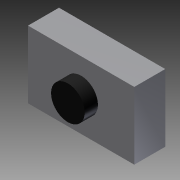
# Autodesk Inventor part: KSR MicroSwitch
Saved by Autodesk Inventor 2012 SP1 (Build 160190100, 190)
## iProperties
Created: 2012-06-05
Part Number: KSR MicroSwitch
Material: Default
Document SubType Name: Modeling
Designer: ding42
Density: 1 g/cm^3
Description: Surface Mount Vertical Tactile Switches
Stock Number: Digi Key Number: 401-1703-1-ND, Manufacturers Number: KSR221GLFS
Catalog Web Link: http://www.digikey.com/catalog/en/partgroup/ksr-series/12817
Author: ding42
Autodesk Inventor part; units mm, degrees
ref_plane "YZ Plane" through (0, 0, 0) normal (1, 0, 0) x (0, 1, 0)
ref_plane "XZ Plane" through (0, 0, 0) normal (0, 1, 0) x (-1, 0, 0)
ref_plane "XY Plane" through (0, 0, 0) normal (0, 0, 1) x (1, 0, 0)
sketch "Sketch1" plane through (0, 0, 0) normal (0, 0, 1) x (1, 0, 0)
  line L0 (0, 0) -> (6, 0)
  line L1 (6, 0) -> (6, -3.8)
  line L2 (6, -3.8) -> (0, -3.8)
  line L3 (0, -3.8) -> (0, 0)
  dimension "d0" = 6
  dimension "d1" = 3.8
  constraints: 8 end point, 2 parallel, 1 horizontal, 1 perpendicular
  measures "d0" distance of L1.end L2.end
  measures "d1" distance of L0.end L1.end
extrude "Extrusion1" add sketch "Sketch1" along normal blind 1.75
sketch "Sketch2" plane through (0, 0, 1.75) normal (0, 0, 1) x (1, 0, 0)
  line L0 (6, 0) -> (6, -3.8) construction
  line L1 (0, 0) -> (6, 0) construction
  line L2 (0, -3.8) -> (0, 0) construction
  line L3 (6, -3.8) -> (0, -3.8) construction
  line L4 (6, -1.9) -> (0, -1.9) construction
  line L5 (3, 0) -> (3, -3.8) construction
  circle A0 centre (3, -1.9) radius 0.95
  dimension "d14" = 1.9
  constraints: 5 midpoint, 4 end point, 1 centre point
  measures "d14" diameter of A0
extrude "Extrusion2" add sketch "Sketch2" along normal blind 0.75
body "Solid1"
